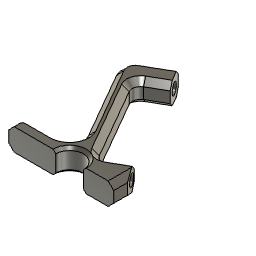
CYD Stand Leg Landscape (Autodesk Fusion 360 design; units mm, degrees)
Autodesk Fusion 360 part; units mm, degrees
sketch "Sketch1" plane through (0, 0, 0) normal (0, 0, 1) x (1, 0, 0)
  line L0 (0, 0) -> (37.9953, 0)
  line L1 (37.9953, 0) -> (37.9953, 5)
  line L2 (12.0145, 5) -> (3, 5)
  line L3 (0, 5) -> (0, 0)
  line L4 (16.3446, 12.5) -> (2.5, 36.4796)
  line L5 (23.5615, 0) -> (125.219, 0) construction
  line L6 (9.8208, 33.7781) -> (24.5459, 8.216)
  line L7 (4.3301, 43.3097) -> (13.0376, 48.3257)
  line L8 (13.0376, 48.3257) -> (17.0308, 41.3935)
  line L9 (17.0308, 41.3935) -> (10.9229, 37.8751)
  line L10 (35.9953, 8.4641) -> (70.9221, 28.5837) construction
  line L11 (15.0342, 44.8596) -> (46.1171, 62.7649) construction
  line L12 (0, 2) -> (0, 0) construction
  line L13 (37.9953, 5) -> (34.7508, 10.6323)
  line L14 (34.7508, 10.6323) -> (28.6429, 7.1139)
  arc A0 (4.3301, 43.3097) -> (2.5, 36.4796) centre (6.8301, 38.9796) ccw
  arc A1 (3, 5) -> (0, 2) centre (3, 2) ccw
  arc A2 (12.0145, 5) -> (16.3446, 12.5) centre (12.0145, 10) ccw
  arc A3 (24.5459, 8.216) -> (28.6429, 7.1139) centre (27.1454, 9.7134) ccw
  arc A4 (10.9229, 37.8751) -> (9.8208, 33.7781) centre (12.4204, 35.2756) ccw
  arc A5 (27.0408, 0) -> (17.0408, 0) centre (22.0408, 0) ccw
  point P0 (0, 40.8097)
  dimension "d1" = 5
  dimension "d2" = 120
  dimension "d3" = 5
  dimension "d4" = 8
  dimension "d6" = 42
  dimension "d9" = 5
  dimension "d10" = 3
  dimension "d11" = 5
  dimension "d12" = 3
  dimension "d13" = 3
  dimension "d24" = 5
  dimension "d30" = 4
  dimension "d31" = 2.5
  constraint horizontal L0
  constraint vertical L1
  constraint horizontal L2
  constraint coincident L0.start L3.end
  constraint horizontal L5
  constraint coincident L0 L5.start
  constraint perpendicular L7 L8
  constraint perpendicular L8 L9
  constraint midpoint L8 L11.start
  constraint perpendicular L8 L11
  constraint perpendicular L6 L9
  constraint coincident L0 L3.end
  constraint perpendicular L0 L12
  constraint collinear L3 L12
  constraint perpendicular L10 L13
  constraint collinear L8 L13
  constraint perpendicular L6 L14
  constraint coincident P0 L4
  constraint tangent L4 A0
  constraint coincident L7.start A0.start
  constraint coincident P0 L12
  constraint coincident L3.start L2
  constraint tangent L12 A1
  constraint tangent L2 A1
  constraint coincident L1.end L2
  constraint coincident L5.start L4
  constraint tangent L2 A2
  constraint tangent L4 A2
  constraint tangent L6 A3
  constraint tangent L14 A3
  constraint coincident L7.start L6
  constraint tangent L9 A4
  constraint tangent L6 A4
  constraint coincident L0 A5.start
  constraint coincident L0 A5.centre
  measures "d1" distance of L0.start L3.start
  measures "d2" angle of L4 L5
  measures "d3" distance of P0 L7.start
  measures "d4" distance of L7.end L8.end
  measures "d6" distance of L10 L11
  measures "d9" radius of A0
  measures "d10" radius of A1
  measures "d11" radius of A2
  measures "d12" radius of A3
  measures "d13" radius of A4
  measures "d24" radius of A5
  measures "d30" distance of L1.end L10
  measures "d31" distance of L10 L14
extrude "Extrude1" add sketch "Sketch1" along normal blind 8 contours L0 L1 L2 L3 L4 L6 L7 L8 L9 L13 L14 A0 A1 A2 A3 A4 A5
sketch "Sketch2" plane through (30.6912, 17.6796, 0) normal (0.866513, 0.499154, 0) x (-0.499154, 0.866513, 0)
  line L0 (27.3671, 0) -> (35.3671, 0)
  line L1 (35.3671, 0) -> (35.3671, 8)
  line L2 (35.3671, 8) -> (27.3671, 8)
  line L3 (27.3671, 8) -> (27.3671, 0)
  line L4 (-14.6329, 0) -> (-8.1329, 0) construction
  line L5 (-8.1329, 0) -> (-8.1329, 8) construction
  line L6 (-8.1329, 8) -> (-14.6329, 8) construction
  line L7 (-14.6329, 8) -> (-14.6329, 0) construction
  line L8 (27.3671, 8) -> (35.3671, 0) construction
  line L9 (35.3671, 8) -> (27.3671, 0) construction
  circle A0 centre (-10.6329, 4) radius 2
  circle A1 centre (31.3671, 4) radius 2
  circle A2 centre (-10.6329, 4) radius 1.6
  circle A3 centre (31.3671, 4) radius 1.6
  line L10 (-10.6329, 8) -> (-10.6329, 0) construction
  dimension "d16" = 4
  dimension "d17" = 4
  dimension "d26" = 3.2
  dimension "d27" = 3.2
  dimension "d32" = 4
  constraint coincident L2.end L3.start
  constraint coincident L0.end L1.start
  constraint coincident L1.end L2.start
  constraint coincident L0.start L3.end
  constraint midpoint L8 A1.centre
  constraint concentric A0 A2
  constraint concentric A1 A3
  constraint coincident L6 L10.start
  constraint coincident L4 L10.end
  constraint perpendicular L4 L10
  constraint midpoint A0.centre L10
  measures "d16" diameter of A0
  measures "d17" diameter of A1
  measures "d26" diameter of A2
  measures "d27" diameter of A3
  measures "d32" distance of L7 L10
extrude "Extrude2" cut sketch "Sketch2" against normal blind 4 contours A0 | A1 | A2 | A3
extrude "Extrude3" cut sketch "Sketch2" against normal blind 10 contours A2 | A3
chamfer "Chamfer1" distance 2 angle 45 26 edges at (7.5073, 5, 8) (16.3446, 7.5, 8) (9.4223, 24.4898, 8) (2.0005, 40.2737, 8) (8.6838, 45.8177, 8) (0, 1, 8) (0.8787, 4.1213, 8) (17.1834, 20.997, 8) (26.3661, 6.8164, 8) (31.6968, 8.8731, 8) (13.9768, 39.6343, 8) (9.5233, 36.0548, 8) (17.1834, 20.997, 0) (9.5233, 36.0548, 0) (13.9768, 39.6343, 0) (31.6968, 8.8731, 0) (26.3661, 6.8164, 0) (9.4223, 24.4898, 0) (16.3446, 7.5, 0) (7.5073, 5, 0) (0.8787, 4.1213, 0) (0, 1, 0) (8.6838, 45.8177, 0) (2.0005, 40.2737, 0) (37.9953, 2.5, 8) (37.9953, 2.5, 0)
chamfer "Chamfer2" distance 1 angle 45 2 edges at (22.0408, 5, 0) (22.0408, 5, 8)
named bodies: "Stand Leg Portrait"
